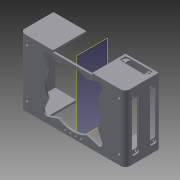
# Autodesk Inventor part: Enclosure03
Saved by Autodesk Inventor 2013 (Build 170138000, 138)
## iProperties
Created: 2014-04-13
Part Number: Enclosure03
Material: Generic
Document SubType Name: Modeling
Designer: spichelh
Density: 1 g/cm^3
Author: spichelh
Autodesk Inventor part; units mm, degrees
ref_plane "YZ Plane" through (0, 0, 0) normal (1, 0, 0) x (0, 1, 0)
ref_plane "XZ Plane" through (0, 0, 0) normal (0, 1, 0) x (-1, 0, 0)
ref_plane "XY Plane" through (0, 0, 0) normal (0, 0, 1) x (1, 0, 0)
sketch "Sketch1" plane through (0, 0, 0) normal (0, 0, 1) x (1, 0, 0)
  circle A0 centre (31.4469, 31.0185) radius 28
  line L0 (-19.3531, 19.1035) -> (82.2469, 19.1035) construction
  line L1 (8.064, 76.2535) -> (-19.3531, 76.2535) construction
  line L2 (82.2469, 76.2535) -> (53.944, 76.2535) construction
  line L3 (82.2469, 19.1035) -> (82.2469, 76.2535) construction
  line L4 (-19.3531, 76.2535) -> (-19.3531, 19.1035) construction
  circle A1 centre (5.126, 22.9135) radius 1.5 construction
  line L5 (5.509, -3.7465) -> (61.389, -3.7465) construction
  line L6 (-22.3531, -3.7465) -> (85.2469, -3.7465)
  line L7 (85.2469, -3.7465) -> (85.2469, 64.2535)
  line L8 (31.4469, -3.7465) -> (31.4469, 78.2535) construction
  circle A2 centre (31.4469, 31.0185) radius 23 projected
  line L9 (-22.3531, 64.2535) -> (-22.3531, -3.7465)
  line L10 (-22.3531, 64.2535) -> (85.2469, 64.2535)
  point P0 (0, 0)
  dimension "d42" = 0
  dimension "d44" = 3
  dimension "d47" = 57.15
  dimension "d49" = 101.6
  dimension "d50" = 3.81
  dimension "d59" = 56
  dimension "d199" = 68
  dimension "d202" = 107.6
  dimension "d374" = 3.7465
  dimension "d375" = 22.3531
  constraints: 22 end point, 2 centre point, 2 parallel, 1 concentric, 1 horizontal, 1 midpoint, 1 perpendicular, 1 point on line, 1 symmetric about line
  measures "d42" distance between parallel lines of L6 L5
  measures "d44" distance between parallel lines of L7 L3
  measures "d47" distance between parallel lines of L0 L1
  measures "d49" distance between parallel lines of L4 L3
  measures "d50" distance from line of L0 A1.centre
  measures "d59" diameter of A0
  measures "d199" distance of L9.start L6.start
  measures "d202" distance between parallel lines of L9 L7
  measures "d374" distance from line of L6 point (0, 0)
  measures "d375" distance from line of L9 point (0, 0)
extrude "Extrusion1" add sketch "Sketch1" along normal blind 2 contours A0 | L9 L10 L7 L6
sketch "Sketch4" plane through (0, 0, 2) normal (0, 0, 1) x (1, 0, 0)
  circle A0 centre (-15.5431, 55.7835) radius 1.5 projected
  circle A1 centre (-15.5431, 6.2535) radius 1.5 projected
  circle A2 centre (78.4369, 6.2535) radius 1.5 projected
  circle A3 centre (78.4369, 55.7835) radius 1.5 projected
  circle A4 centre (-15.5431, 55.7835) radius 1.4
  circle A5 centre (-15.5431, 6.2535) radius 1.4
  circle A6 centre (78.4369, 6.2535) radius 1.4
  circle A7 centre (78.4369, 55.7835) radius 1.4
  point P0 (0, 0)
  dimension "d490" = 2.8
  dimension "d491" = 2.8
  dimension "d492" = 2.8
  dimension "d493" = 2.8
  constraints: 4 centre point, 4 coincident
  measures "d490" diameter of A4
  measures "d491" diameter of A5
  measures "d492" diameter of A6
  measures "d493" diameter of A7
extrude "Extrusion3" cut sketch "Sketch4" against normal blind 10 contours A4 | A5 | A6 | A7
sketch "Sketch2" plane through (0, 0, 0) normal (0, 0, -1) x (-1, 0, 0)
  circle A0 centre (-31.4469, 31.0185) radius 23 projected
  line L0 (20.3531, 62.2535) -> (20.3531, -1.7465)
  line L1 (20.3531, -1.7465) -> (-83.2469, -1.7465)
  line L2 (-83.2469, -1.7465) -> (-83.2469, 62.2535)
  line L3 (-83.2469, 62.2535) -> (20.3531, 62.2535)
  circle A1 centre (-31.4469, 31.0185) radius 23 projected
  line L4 (22.3531, -3.7465) -> (-85.2469, -3.7465) projected
  line L5 (22.3531, 64.2535) -> (22.3531, -3.7465) projected
  line L6 (-85.2469, 64.2535) -> (22.3531, 64.2535) projected
  line L7 (-85.2469, -3.7465) -> (-85.2469, 64.2535) projected
  dimension "d454" = 2
  dimension "d455" = 2
  dimension "d456" = 2
  dimension "d457" = 2
  constraints: 8 end point
  measures "d454" distance between parallel lines of L6 L3
  measures "d455" distance between parallel lines of L5 L0
  measures "d456" distance between parallel lines of L4 L1
  measures "d457" distance between parallel lines of L7 L2
extrude "Extrusion2" add sketch "Sketch2" along normal blind 32 contours L4 L7 L6 L5
ref_plane "Work Plane1" through (0, 0, 7) normal (0, 0, -1) x (-1, 0, 0)
sketch "Sketch28" plane through (0, 0, 7) normal (0, 0, -1) x (-1, 0, 0)
  circle A0 centre (-31.4469, 31.0185) radius 28 projected
  circle A1 centre (-31.4469, 31.0185) radius 31
  point P0 (0, 0)
  dimension "d209" = 62
  constraints: 1 centre point, 1 coincident
  measures "d209" diameter of A1
extrude "Extrusion23" [suppressed]
sketch "Sketch5" plane through (-22.3531, 77.2535, 10) normal (0, 1, 0) x (-0.9933511, 0, -0.1151242)
  line L0 (0, 0) -> (128.1647, 0)
  line L1 (36.0824, 63) -> (92.0824, 63)
  line L2 (92.0824, 63) -> (92.0824, 7)
  line L3 (92.0824, 7) -> (36.0824, 7)
  line L4 (36.0824, 7) -> (36.0824, 63)
  line L5 (64.0824, 0) -> (64.0824, -31.7336) construction
  line L6 (36.0824, 63) -> (92.0824, 7) construction
  line L7 (92.0824, 63) -> (36.0824, 7) construction
  line L8 (104.9242, 0) -> (-0.6758, 0)
  line L9 (-53.8, -48) -> (-9.5691, -16.8574) construction
  point P0 (19.351, -30)
  point P1 (64.0824, 35)
  point P2 (64.0824, 35)
  dimension "d28" = 56
  dimension "d29" = 56
  dimension "d41" = 7
  constraints: 20 end point, 3 midpoint, 3 parallel, 2 point on line, 1 collinear, 1 horizontal, 1 perpendicular
  measures "d28" distance of L2.end L3.end
  measures "d29" distance of L1.end L2.end
  measures "d41" distance between parallel lines of L8 L3
extrude "Extrusion4" [suppressed]
sketch "Sketch6" plane through (-6.7798, 80.573, 3) normal (0, 1, 0) x (1, 0, 0)
  line L0 (71.5763, -7) -> (-25.8, -7) projected
  line L1 (0, 0) -> (56, 0)
  line L2 (56, 0) -> (56, -7)
  line L3 (56, -7) -> (0, -7)
  line L4 (0, -7) -> (0, 0)
  point P0 (76.8, -7)
  point P1 (-20.8, -7)
  point P2 (6.7798, 3)
  point P3 (71.5763, -8)
  point P4 (-25.8, -7)
  constraints: 8 end point, 2 parallel, 1 horizontal, 1 perpendicular, 2 other
extrude "Extrusion5" [suppressed]
sketch "Sketch7" plane through (0, 0, 2) normal (0, 0, 1) x (1, 0, 0)
  line L0 (-22.3531, -3.7465) -> (85.2469, -3.7465) projected
  line L1 (59.4469, 75.7535) -> (3.4469, 75.7535) projected
  line L2 (31.4469, -3.7465) -> (31.4469, 75.7535) construction
  line L3 (23.1969, -0.7465) -> (23.1969, -0.7465)
  line L4 (22.1969, 0.2535) -> (22.1969, 1.2535)
  line L5 (23.1969, 2.2535) -> (23.1969, 2.2535)
  line L6 (24.1969, 1.2535) -> (24.1969, 0.2535)
  arc A0 (24.1969, 1.2535) -> (23.1969, 2.2535) centre (23.1969, 1.2535) ccw
  arc A1 (23.1969, 2.2535) -> (22.1969, 1.2535) centre (23.1969, 1.2535) ccw
  arc A2 (22.1969, 0.2535) -> (23.1969, -0.7465) centre (23.1969, 0.2535) ccw
  arc A3 (23.1969, -0.7465) -> (24.1969, 0.2535) centre (23.1969, 0.2535) ccw
  line L7 (27.6969, 0.2535) -> (27.6969, 1.2535)
  line L8 (29.6969, 1.2535) -> (29.6969, 0.2535)
  arc A4 (29.6969, 1.2535) -> (28.6969, 2.2535) centre (28.6969, 1.2535) ccw
  arc A5 (28.6969, 2.2535) -> (27.6969, 1.2535) centre (28.6969, 1.2535) ccw
  arc A6 (27.6969, 0.2535) -> (28.6969, -0.7465) centre (28.6969, 0.2535) ccw
  arc A7 (28.6969, -0.7465) -> (29.6969, 0.2535) centre (28.6969, 0.2535) ccw
  line L9 (33.1969, 0.2535) -> (33.1969, 1.2535)
  line L10 (35.1969, 1.2535) -> (35.1969, 0.2535)
  arc A8 (35.1969, 1.2535) -> (34.1969, 2.2535) centre (34.1969, 1.2535) ccw
  arc A9 (34.1969, 2.2535) -> (33.1969, 1.2535) centre (34.1969, 1.2535) ccw
  arc A10 (33.1969, 0.2535) -> (34.1969, -0.7465) centre (34.1969, 0.2535) ccw
  arc A11 (34.1969, -0.7465) -> (35.1969, 0.2535) centre (34.1969, 0.2535) ccw
  line L11 (38.6969, 0.2535) -> (38.6969, 1.2535)
  line L12 (40.6969, 1.2535) -> (40.6969, 0.2535)
  arc A12 (40.6969, 1.2535) -> (39.6969, 2.2535) centre (39.6969, 1.2535) ccw
  arc A13 (39.6969, 2.2535) -> (38.6969, 1.2535) centre (39.6969, 1.2535) ccw
  arc A14 (38.6969, 0.2535) -> (39.6969, -0.7465) centre (39.6969, 0.2535) ccw
  arc A15 (39.6969, -0.7465) -> (40.6969, 0.2535) centre (39.6969, 0.2535) ccw
  line L13 (29.6969, 0.7535) -> (33.1969, 0.7535) construction
  point P0 (-17.3531, -3.7465)
  point P1 (80.2469, -3.7465)
  point P2 (0, 0)
  point P3 (24.1969, -0.7465)
  point P4 (22.1969, 2.2535)
  point P5 (24.1969, 2.2535)
  point P6 (29.6969, -0.7465)
  point P7 (27.6969, 2.2535)
  point P8 (29.6969, 2.2535)
  point P9 (35.1969, -0.7465)
  point P10 (33.1969, 2.2535)
  point P11 (35.1969, 2.2535)
  point P12 (40.6969, -0.7465)
  point P13 (38.6969, 2.2535)
  point P14 (40.6969, 2.2535)
  point P15 (31.4469, 0.7535)
  dimension "d64" = 2
  dimension "d66" = 3
  dimension "d67" = 1
  dimension "d68" = 1
  dimension "d69" = 4
  dimension "d78" = 16.5
  dimension "d79" = 7.25
  dimension "d80" = 7.25
  constraints: 32 point on circle, 24 end point, 16 centre point, 16 point on line, 8 tangent, 5 midpoint, 2 equal radius, 2 parallel, 1 horizontal, 1 perpendicular
  measures "d64" distance of point (22.197, 2.253) point (24.197, 2.253)
  measures "d66" distance of point (24.197, 2.253) point (24.197, -0.747)
  measures "d67" radius of A0
  measures "d68" radius of A3
  measures "d69" distance from line of L0 A3.centre
  measures "d78" distance of A14.centre A3.centre
  measures "d79" distance from line of L6 point (31.447, 0.753)
  measures "d80" distance from line of point (31.447, 0.753) L11
extrude "Extrusion6" cut sketch "Sketch7" against normal blind 5
sketch "Sketch42" plane through (0, 0, 2) normal (0, 0, 1) x (1, 0, 0)
  circle A0 centre (31.4469, 31.0185) radius 28 projected
  arc A1 (33.1969, 0.2535) -> (35.1969, 0.2535) centre (34.1969, 0.2535) ccw projected
  line L0 (33.1969, 0.2535) -> (33.1969, 1.2535) projected
  arc A2 (35.1969, 1.2535) -> (33.1969, 1.2535) centre (34.1969, 1.2535) ccw projected
  line L1 (35.1969, 1.2535) -> (35.1969, 0.2535) projected
  arc A3 (33.1969, 0.2535) -> (35.1969, 0.2535) centre (34.1969, 0.2535) ccw projected
  circle A4 centre (31.4469, 27.6995) radius 31 projected
  line L2 (38.6969, 0.2535) -> (38.6969, 1.2535) projected
  arc A5 (40.6969, 1.2535) -> (38.6969, 1.2535) centre (39.6969, 1.2535) ccw projected
  circle A6 centre (31.4469, 27.6995) radius 31 projected
  arc A7 (24.1969, 1.2535) -> (22.1969, 1.2535) centre (23.1969, 1.2535) ccw projected
  line L3 (24.1969, 1.2535) -> (24.1969, 0.2535) projected
  circle A8 centre (31.4469, 27.6995) radius 31 projected
  arc A9 (27.6969, 0.2535) -> (29.6969, 0.2535) centre (28.6969, 0.2535) ccw projected
  line L4 (27.6969, 0.2535) -> (27.6969, 1.2535) projected
  arc A10 (29.6969, 1.2535) -> (27.6969, 1.2535) centre (28.6969, 1.2535) ccw projected
  line L5 (29.6969, 1.2535) -> (29.6969, 0.2535) projected
  arc A11 (27.6969, 0.2535) -> (29.6969, 0.2535) centre (28.6969, 0.2535) ccw projected
  circle A12 centre (31.4469, 27.6995) radius 31 projected
  point P0 (33.214, 0.0694)
  point P1 (35.1969, 0.2466)
  point P2 (38.6969, 0.8787)
  point P3 (40.6819, 1.4265)
  point P4 (22.212, 1.4265)
  point P5 (24.1969, 0.8787)
  point P6 (27.697, 0.2466)
  point P7 (29.6799, 0.0694)
  point P8 (0, 0)
  point P9 (33.2141, 0.0689)
  point P10 (35.1969, 0.2461)
  point P11 (38.6969, 0.8782)
  point P12 (40.6819, 1.426)
  point P13 (22.2119, 1.426)
  point P14 (24.1969, 0.8782)
  point P15 (27.697, 0.2461)
  point P16 (29.6798, 0.0689)
  constraints: 1 coincident, 4 other
sketch "Sketch43" plane through (0, 0, 2) normal (0, 0, 1) x (1, 0, 0)
  circle A0 centre (4.7769, 55.7835) radius 1.4
  arc A1 (5.8515, 59.1144) -> (1.5346, 54.4655) centre (4.7769, 55.7835) ccw
  circle A2 centre (31.4469, 31.0185) radius 20
  line L0 (5.8515, 59.1144) -> (16.9262, 55.5419)
  line L1 (1.5346, 54.4655) -> (5.9166, 43.6854)
  circle A3 centre (4.7769, 6.2535) radius 1.4
  circle A4 centre (58.1169, 6.2535) radius 1.4
  line L2 (58.1169, 55.7835) -> (4.7769, 6.2535) construction
  line L3 (58.1169, 6.2535) -> (4.7769, 55.7835) construction
  line L4 (31.4469, 31.0185) -> (31.4469, 40.8752) construction
  line L5 (31.4469, 31.0185) -> (19.6856, 31.0185) construction
  line L6 (57.0424, 59.1144) -> (45.9677, 55.5419)
  arc A5 (61.3593, 54.4655) -> (57.0424, 59.1144) centre (58.1169, 55.7835) ccw
  line L7 (61.3593, 54.4655) -> (56.9773, 43.6854)
  circle A6 centre (58.1169, 55.7835) radius 1.4
  arc A7 (45.9677, 55.5419) -> (16.9262, 55.5419) centre (31.4469, 31.0185) ccw
  arc A8 (5.9166, 43.6854) -> (56.9773, 43.6854) centre (31.4469, 31.0185) ccw construction
  arc A9 (45.9677, 55.5419) -> (16.9262, 55.5419) centre (31.4469, 31.0185) ccw construction
  arc A10 (1.5346, 7.5715) -> (5.8515, 2.9225) centre (4.7769, 6.2535) ccw
  line L8 (5.8515, 2.9225) -> (16.9262, 6.495)
  line L9 (1.5346, 7.5715) -> (5.9166, 18.3516)
  line L10 (61.3593, 7.5715) -> (56.9773, 18.3516)
  arc A11 (57.0424, 2.9225) -> (61.3593, 7.5715) centre (58.1169, 6.2535) ccw
  line L11 (57.0424, 2.9225) -> (45.9677, 6.495)
  arc A12 (56.9773, 18.3516) -> (56.9773, 43.6854) centre (31.4469, 31.0185) ccw
  arc A13 (5.9166, 43.6854) -> (5.9166, 18.3516) centre (31.4469, 31.0185) ccw
  arc A14 (16.9262, 6.495) -> (45.9677, 6.495) centre (31.4469, 31.0185) ccw
  circle A15 centre (31.4469, 31.0185) radius 28 projected
  line L12 (85.2469, -1.7465) -> (85.2469, 65.2535) construction
  line L13 (85.2469, 65.2535) -> (54.4469, 65.2535) construction
  line L14 (8.4469, 65.2535) -> (-22.3531, 65.2535) construction
  line L15 (-22.3531, 65.2535) -> (-22.3531, -1.7465) construction
  line L16 (-20.3531, -3.7465) -> (83.2469, -3.7465) construction
  line L17 (85.2469, 65.2535) -> (-22.0418, -2.818) construction
  line L18 (-22.3531, 65.2535) -> (84.9357, -2.818) construction
  point P0 (3.5014, 0.0834)
  point P1 (31.4469, 31.0185)
  point P2 (67.9135, 65.2535)
  point P3 (-5.0196, 65.2535)
  point P4 (-10.4012, -3.7465)
  point P5 (73.2951, -3.7465)
  dimension "d345" = 2.8
  dimension "d346" = 7
  dimension "d347" = 40
  dimension "d348" = 27.9456
  dimension "d349" = 53.34
  dimension "d350" = 49.53
  dimension "d351" = 2.8
  dimension "d352" = 2.8
  dimension "d353" = 155
  dimension "d354" = 155
  dimension "d355" = 30.9351
  dimension "d356" = 28.5
  dimension "d357" = 155
  dimension "d358" = 3.5
  dimension "d359" = 155
  dimension "d360" = 28.5
  constraints: 28 end point, 22 point on circle, 15 centre point, 10 symmetric about line, 7 coincident, 4 tangent, 2 horizontal alignment, 2 midpoint, 2 vertical alignment, 1 perpendicular, 9 other
  measures "d345" diameter of A0
  measures "d346" diameter of A1
  measures "d347" diameter of A2
  measures "d348" horizontal distance of L4.start point (3.501, 0.083)
  measures "d349" distance of A0.centre L2.start
  measures "d350" distance of point (4.777, 6.253) A0.centre
  measures "d351" diameter of A3
  measures "d352" diameter of A4
  measures "d353" angle of L3 L0
  measures "d354" angle of L3 L1
  measures "d355" vertical distance of point (3.501, 0.083) A8.centre
  measures "d356" radius of A7
  measures "d357" angle of L8 L2
  measures "d358" radius of A10
  measures "d359" angle of L2 L9
  measures "d360" radius of A12
extrude "Extrusion32" cut sketch "Sketch43" against normal blind 10 contours A0 | L0 A7 L6 A5 L7 A12 L10 A11 L11 A14 L8 A10 L9 A13 L1 A1 | A3 | A4 | A6 | A15
sketch "Sketch44" plane through (85.2469, -3.7465, 2) normal (1, 0, 0) x (0, 0, -1)
  line L0 (9, 56.4) -> (12, 56.4)
  line L1 (14, 54.4) -> (14, 13.4)
  line L2 (12, 11.4) -> (9, 11.4)
  line L3 (7, 13.4) -> (7, 54.4)
  line L4 (10.671, 0) -> (39, 0)
  arc A0 (14, 54.4) -> (12, 56.4) centre (12, 54.4) ccw
  arc A1 (9, 56.4) -> (7, 54.4) centre (9, 54.4) ccw
  arc A2 (12, 11.4) -> (14, 13.4) centre (12, 13.4) ccw
  arc A3 (7, 13.4) -> (9, 11.4) centre (9, 13.4) ccw
  line L5 (0, 0) -> (0, 68) projected
  line L6 (34, 0) -> (0, 0) projected
  line L7 (34, 68) -> (0, 68) projected
  line L8 (0, 0) -> (0, 68) projected
  line L9 (34, 0) -> (0, 0) projected
  line L10 (34, 68) -> (34, 0) projected
  point P0 (-28, 1.7465)
  point P1 (7, 56.4)
  point P2 (14, 56.4)
  point P3 (-39, 45.4825)
  point P4 (-57, 11.6532)
  point P5 (0, 15.1877)
  point P6 (0, 0)
  dimension "d310" = 45
  dimension "d312" = 7
  dimension "d313" = 11.4
  dimension "d314" = 7
  dimension "d315" = 2
  dimension "d483" = 11.6
  constraints: 10 end point, 8 point on circle, 8 tangent, 5 point on line, 4 centre point, 3 equal radius, 2 parallel, 1 collinear, 1 horizontal, 1 perpendicular, 4 other
  measures "d310" distance between parallel lines of L0 L2
  measures "d312" distance of point (7, 56.4) point (14, 56.4)
  measures "d313" distance between parallel lines of L4 L2
  measures "d314" distance of the line from the sketch origin of L3
  measures "d315" radius of A0
  measures "d483" distance between parallel lines of L7 L0
extrude "Extrusion33" cut sketch "Sketch44" against normal blind 50 contours L0 A0 L1 A2 L2 A3 L3 A1
sketch "Sketch45" plane through (85.2469, -3.7465, 2) normal (1, 0, 0) x (0, 0, -1)
  arc A0 (9, 56.4) -> (7, 54.4) centre (9, 54.4) ccw
  line L0 (9, 56.4) -> (12, 56.4)
  arc A1 (14, 54.4) -> (12, 56.4) centre (12, 54.4) ccw
  line L1 (14, 54.4) -> (14, 13.4)
  arc A2 (12, 11.4) -> (14, 13.4) centre (12, 13.4) ccw
  line L2 (12, 11.4) -> (9, 11.4)
  arc A3 (7, 13.4) -> (9, 11.4) centre (9, 13.4) ccw
  line L3 (7, 13.4) -> (7, 54.4)
  line L4 (9, 60.4) -> (12, 60.4)
  line L5 (14, 58.4) -> (14, 9.4)
  line L6 (12, 7.4) -> (9, 7.4)
  line L7 (7, 9.4) -> (7, 58.4)
  arc A4 (14, 58.4) -> (12, 60.4) centre (12, 58.4) ccw
  arc A5 (9, 60.4) -> (7, 58.4) centre (9, 58.4) ccw
  arc A6 (12, 7.4) -> (14, 9.4) centre (12, 9.4) ccw
  arc A7 (7, 9.4) -> (9, 7.4) centre (9, 9.4) ccw
  arc A8 (9, 56.4) -> (7, 54.4) centre (9, 54.4) ccw projected
  line L8 (9, 56.4) -> (12, 56.4) projected
  line L9 (12, 11.4) -> (9, 11.4) projected
  arc A9 (7, 13.4) -> (9, 11.4) centre (9, 13.4) ccw projected
  line L10 (7, 13.4) -> (7, 54.4) projected
  arc A10 (14, 54.4) -> (12, 56.4) centre (12, 54.4) ccw projected
  line L11 (14, 54.4) -> (14, 13.4) projected
  arc A11 (12, 11.4) -> (14, 13.4) centre (12, 13.4) ccw projected
  point P0 (-28, 1.7465)
  point P1 (-29.2165, 54.9882)
  point P2 (-29.1727, 10.0075)
  dimension "d485" = 2
  dimension "d487" = 2
  dimension "d330" = 0
  dimension "d331" = 4
  dimension "d332" = 4
  dimension "d333" = 0
  dimension "d334" = 2
  dimension "d484" = 2
  dimension "d486" = 2
  dimension "d488" = 2
  constraints: 16 end point, 12 point on circle, 8 tangent, 6 centre point, 4 coincident, 4 collinear, 3 equal radius, 2 parallel, 1 horizontal, 1 perpendicular, 8 other
  measures "d330" distance between parallel lines of L5 L1
  measures "d331" distance between parallel lines of L4 L0
  measures "d332" distance between parallel lines of L2 L6
  measures "d333" distance between parallel lines of L3 L7
  measures "d334" radius of A4
  measures "d484" radius of A2
  measures "d486" radius of A6
  measures "d488" radius of A1
extrude "Extrusion34" cut sketch "Sketch45" against normal blind 1.5 contours A0 L7 A5 L4 A4 L5 A1 L0 | A3 L2 A2 L5 A6 L6 A7 L7
sketch "Sketch46" plane through (85.2469, -3.7465, 2) normal (1, 0, 0) x (0, 0, -1)
  line L0 (12, 56.4) -> (9, 56.4)
  line L1 (-25, 13.4) -> (-25, 54.4)
  arc A0 (9, 60.4) -> (7, 58.4) centre (9, 58.4) ccw
  line L2 (14, 58.4) -> (14, 9.4)
  circle A1 centre (9, 58.4) radius 1
  line L3 (9, 58.4) -> (7.5858, 59.8142) construction
  line L4 (10.5, 56.4) -> (10.5, 46.2799) construction
  circle A2 centre (12, 58.4) radius 1
  line L5 (-25, 33.9) -> (-40, 33.9) construction
  circle A3 centre (9, 9.4) radius 1
  circle A4 centre (12, 9.4) radius 1
  line L6 (12, 56.4) -> (9, 56.4) projected
  arc A5 (9, 60.4) -> (7, 58.4) centre (9, 58.4) ccw projected
  arc A6 (12, 7.4) -> (14, 9.4) centre (12, 9.4) ccw projected
  point P0 (2, 3.7465)
  point P1 (-29.1529, 58.9941)
  dimension "d337" = 2
  dimension "d340" = 0
  constraints: 12 end point, 4 centre point, 3 symmetric about line, 2 coincident, 2 midpoint, 1 collinear, 1 parallel, 1 perpendicular, 1 point on line, 8 other
  measures "d337" diameter of A1
  measures "d340" distance of L3.start A1.centre
extrude "Extrusion35" cut sketch "Sketch46" against normal blind 2 contours A1 | A4
fillet "Fillet12" radius 0.2 9 edges at (59.1683, 49.0754, 2) (59.9469, 31.0185, 2) (59.1683, 12.9615, 2) (31.4469, 2.5185, 2) (51.505, 4.7088, 2) (11.3888, 4.7088, 2) (3.7256, 12.9615, 2) (2.9469, 31.0185, 2) (3.7256, 49.0754, 2)
fillet "Fillet13" radius 0.2 14 edges at (85.2469, 4.2393, -11.4142) (85.2469, 3.6535, -8.5) (85.2469, 4.2393, -5.5858) (85.2469, 30.1535, -5) (85.2469, 56.0677, -5.5858) (85.2469, 56.6535, -8.5) (85.2469, 56.0677, -11.4142) (85.2469, 30.1535, -12) (83.7469, 52.0677, -11.4142) (83.7469, 52.6535, -8.5) (83.7469, 52.0677, -5.5858) (83.7469, 8.2393, -5.5858) (83.7469, 7.6535, -8.5) (83.7469, 8.2393, -11.4142)
sketch "Sketch50" plane through (85.2469, -3.7465, 2) normal (1, 0, 0) x (0, 0, -1)
  line L0 (0, 68) -> (-34.1358, 68)
  line L1 (0, 8) -> (0, 57)
  line L2 (27.2, 56.3) -> (30.2, 56.3)
  line L3 (32.2, 54.3) -> (32.2, 13.3)
  line L4 (30.2, 11.3) -> (27.2, 11.3)
  line L5 (25.2, 13.3) -> (25.2, 54.3)
  arc A0 (32.2, 54.3) -> (30.2, 56.3) centre (30.2, 54.3) ccw
  arc A1 (27.2, 56.3) -> (25.2, 54.3) centre (27.2, 54.3) ccw
  arc A2 (30.2, 11.3) -> (32.2, 13.3) centre (30.2, 13.3) ccw
  arc A3 (25.2, 13.3) -> (27.2, 11.3) centre (27.2, 13.3) ccw
  line L6 (34, 68) -> (0, 68) projected
  line L7 (0, 0) -> (0, 68) projected
  line L8 (34, 68) -> (34, 0) projected
  point P0 (0, 68)
  point P1 (-34.1358, 68)
  point P2 (-28, 1.7465)
  point P3 (25.2, 56.3)
  point P4 (32.2, 56.3)
  point P5 (-28.0348, 67)
  point P6 (-34, 67)
  dimension "d400" = 45
  dimension "d401" = 7
  dimension "d402" = 2
  dimension "d404" = 11.7
  dimension "d478" = 1.8
  constraints: 10 end point, 8 point on circle, 8 tangent, 4 centre point, 4 point on line, 3 equal radius, 2 horizontal, 2 parallel, 1 collinear, 1 perpendicular, 3 other
  measures "d400" distance between parallel lines of L2 L4
  measures "d401" distance of point (25.2, 56.3) point (32.2, 56.3)
  measures "d402" radius of A0
  measures "d478" distance between parallel lines of L3 L8
extrude "Extrusion39" cut sketch "Sketch50" against normal blind 5
sketch "Sketch51" plane through (85.2469, -3.7465, 2) normal (1, 0, 0) x (0, 0, -1)
  arc A0 (32.2, 54.3) -> (30.2, 56.3) centre (30.2, 54.3) ccw
  line L0 (32.2, 54.3) -> (32.2, 13.3)
  arc A1 (30.2, 11.3) -> (32.2, 13.3) centre (30.2, 13.3) ccw
  line L1 (30.2, 11.3) -> (27.2, 11.3)
  arc A2 (25.2, 13.3) -> (27.2, 11.3) centre (27.2, 13.3) ccw
  line L2 (25.2, 13.3) -> (25.2, 54.3)
  arc A3 (27.2, 56.3) -> (25.2, 54.3) centre (27.2, 54.3) ccw
  line L3 (27.2, 56.3) -> (30.2, 56.3)
  line L4 (27.2, 60.3) -> (30.2, 60.3)
  line L5 (32.2, 58.3) -> (32.2, 9.3)
  line L6 (30.2, 7.3) -> (27.2, 7.3)
  line L7 (25.2, 9.3) -> (25.2, 58.3)
  arc A4 (32.2, 58.3) -> (30.2, 60.3) centre (30.2, 58.3) ccw
  arc A5 (27.2, 60.3) -> (25.2, 58.3) centre (27.2, 58.3) ccw
  arc A6 (30.2, 7.3) -> (32.2, 9.3) centre (30.2, 9.3) ccw
  arc A7 (25.2, 9.3) -> (27.2, 7.3) centre (27.2, 9.3) ccw
  arc A8 (32.2, 54.3) -> (30.2, 56.3) centre (30.2, 54.3) ccw projected
  line L8 (30.2, 11.3) -> (27.2, 11.3) projected
  arc A9 (25.2, 13.3) -> (27.2, 11.3) centre (27.2, 13.3) ccw projected
  line L9 (25.2, 13.3) -> (25.2, 54.3) projected
  arc A10 (27.2, 56.3) -> (25.2, 54.3) centre (27.2, 54.3) ccw projected
  line L10 (27.2, 56.3) -> (30.2, 56.3) projected
  line L11 (32.2, 54.3) -> (32.2, 13.3) projected
  arc A11 (30.2, 11.3) -> (32.2, 13.3) centre (30.2, 13.3) ccw projected
  point P0 (-28, 1.7465)
  point P1 (0, 53.833)
  point P2 (0, 9.167)
  dimension "d480" = 2
  dimension "d482" = 2
  dimension "d411" = 2
  dimension "d412" = 4
  dimension "d413" = 4
  dimension "d415" = 0
  dimension "d479" = 2
  dimension "d481" = 2
  constraints: 16 end point, 12 point on circle, 8 tangent, 6 centre point, 5 collinear, 4 coincident, 3 equal radius, 2 parallel, 1 horizontal, 1 perpendicular, 1 vertical, 8 other
  measures "d411" radius of A4
  measures "d412" distance between parallel lines of L6 L1
  measures "d413" distance between parallel lines of L4 L3
  measures "d415" distance between parallel lines of L2 L7
  measures "d479" radius of A3
  measures "d481" radius of A2
extrude "Extrusion40" cut sketch "Sketch51" against normal blind 1.5 contours A0 L3 A3 L7 A5 L4 A4 L5 | L5 A6 L6 A7 L7 A2 L1 A1
fillet "Fillet16" radius 0.2 14 edges at (85.2469, 4.1393, -29.6142) (85.2469, 3.5535, -26.7) (85.2469, 4.1393, -23.7858) (85.2469, 30.0535, -23.2) (85.2469, 55.9677, -23.7858) (85.2469, 56.5535, -26.7) (85.2469, 55.9677, -29.6142) (85.2469, 30.0535, -30.2) (83.7469, 52.5535, -26.7) (83.7469, 51.9677, -23.7858) (83.7469, 8.1393, -23.7858) (83.7469, 7.5535, -26.7) (83.7469, 8.1393, -29.6142) (83.7469, 51.9677, -29.6142)
sketch "Sketch52" plane through (83.7469, -3.7465, 2) normal (1, 0, 0) x (0, 0, -1)
  arc A0 (30.2, 7.3) -> (32.2, 9.3) centre (30.2, 9.3) ccw projected
  arc A1 (27.2, 60.3) -> (25.2, 58.3) centre (27.2, 58.3) ccw projected
  circle A2 centre (27.2, 58.3) radius 1
  circle A3 centre (30.2, 9.3) radius 1
  point P0 (2, 3.7465)
  dimension "d419" = 2
  dimension "d420" = 2
  constraints: 2 centre point, 2 coincident
  measures "d419" diameter of A2
  measures "d420" diameter of A3
extrude "Extrusion41" cut sketch "Sketch52" against normal blind 2
sketch "Sketch53" plane through (-22.3531, 64.2535, 2) normal (0, 1, 0) x (1, 0, 0)
  line L0 (82.1, 32.2) -> (98.1, 32.2)
  line L1 (100.1, 30.2) -> (100.1, 27.2)
  line L2 (98.1, 25.2) -> (82.1, 25.2)
  line L3 (80.1, 27.2) -> (80.1, 30.2)
  arc A0 (82.1, 32.2) -> (80.1, 30.2) centre (82.1, 30.2) ccw
  arc A1 (80.1, 27.2) -> (82.1, 25.2) centre (82.1, 27.2) ccw
  arc A2 (98.1, 25.2) -> (100.1, 27.2) centre (98.1, 27.2) ccw
  arc A3 (100.1, 30.2) -> (98.1, 32.2) centre (98.1, 30.2) ccw
  line L4 (107.6, 34) -> (107.6, 0) projected
  line L5 (0, 34) -> (107.6, 34) projected
  point P0 (-54.4469, -28)
  point P1 (30.8, -28.0348)
  point P2 (30.8, -34)
  dimension "d423" = 7
  dimension "d425" = 2
  dimension "d426" = 20
  dimension "d460" = 7.5
  dimension "d467" = 1.8
  constraints: 8 end point, 8 point on circle, 8 tangent, 4 centre point, 3 equal radius, 2 parallel, 1 horizontal, 1 perpendicular
  measures "d423" distance between parallel lines of L2 L0
  measures "d425" radius of A0
  measures "d426" distance between parallel lines of L3 L1
  measures "d460" distance between parallel lines of L1 L4
  measures "d467" distance between parallel lines of L5 L0
extrude "Extrusion42" cut sketch "Sketch53" against normal blind 10
sketch "Sketch54" plane through (-22.3531, 64.2535, 2) normal (0, 1, 0) x (1, 0, 0)
  arc A0 (82.1, 32.2) -> (80.1, 30.2) centre (82.1, 30.2) ccw
  line L0 (82.1, 32.2) -> (98.1, 32.2)
  arc A1 (100.1, 30.2) -> (98.1, 32.2) centre (98.1, 30.2) ccw
  line L1 (100.1, 30.2) -> (100.1, 27.2)
  arc A2 (98.1, 25.2) -> (100.1, 27.2) centre (98.1, 27.2) ccw
  line L2 (98.1, 25.2) -> (82.1, 25.2)
  arc A3 (80.1, 27.2) -> (82.1, 25.2) centre (82.1, 27.2) ccw
  line L3 (80.1, 27.2) -> (80.1, 30.2)
  line L4 (78.1, 32.2) -> (102.1, 32.2)
  line L5 (104.1, 30.2) -> (104.1, 27.2)
  line L6 (102.1, 25.2) -> (78.1, 25.2)
  line L7 (76.1, 27.2) -> (76.1, 30.2)
  arc A4 (104.1, 30.2) -> (102.1, 32.2) centre (102.1, 30.2) ccw
  arc A5 (102.1, 25.2) -> (104.1, 27.2) centre (102.1, 27.2) ccw
  arc A6 (76.1, 27.2) -> (78.1, 25.2) centre (78.1, 27.2) ccw
  arc A7 (78.1, 32.2) -> (76.1, 30.2) centre (78.1, 30.2) ccw
  arc A8 (82.1, 32.2) -> (80.1, 30.2) centre (82.1, 30.2) ccw projected
  line L8 (82.1, 32.2) -> (98.1, 32.2) projected
  arc A9 (100.1, 30.2) -> (98.1, 32.2) centre (98.1, 30.2) ccw projected
  line L9 (100.1, 30.2) -> (100.1, 27.2) projected
  arc A10 (98.1, 25.2) -> (100.1, 27.2) centre (98.1, 27.2) ccw projected
  line L10 (98.1, 25.2) -> (82.1, 25.2) projected
  arc A11 (80.1, 27.2) -> (82.1, 25.2) centre (82.1, 27.2) ccw projected
  line L11 (80.1, 27.2) -> (80.1, 30.2) projected
  point P0 (-54.4469, -28)
  dimension "d431" = 2
  dimension "d432" = 4
  dimension "d433" = 4
  dimension "d462" = 2
  dimension "d463" = 2
  dimension "d464" = 2
  dimension "d465" = 2
  constraints: 16 end point, 16 point on circle, 8 centre point, 8 tangent, 6 collinear, 4 coincident, 3 equal radius, 2 horizontal, 2 parallel, 1 perpendicular
  measures "d431" radius of A4
  measures "d432" distance between parallel lines of L1 L5
  measures "d433" distance between parallel lines of L3 L7
  measures "d462" radius of A1
  measures "d463" radius of A3
  measures "d464" radius of A0
  measures "d465" radius of A2
extrude "Extrusion43" cut sketch "Sketch54" against normal blind 1.5 contours A0 L3 A3 L6 A6 L7 A7 L4 | L4 A4 L5 A5 L6 A2 L1 A1
sketch "Sketch55" plane through (-22.3531, 62.7535, 2) normal (0, 1, 0) x (1, 0, 0)
  arc A0 (104.1, 30.2) -> (102.1, 32.2) centre (102.1, 30.2) ccw projected
  circle A1 centre (102.1, 30.2) radius 1
  arc A2 (80.1, 27.2) -> (82.1, 25.2) centre (82.1, 27.2) ccw projected
  line L0 (80.1, 30.2) -> (80.1, 27.2) projected
  arc A3 (82.1, 32.2) -> (80.1, 30.2) centre (82.1, 30.2) ccw projected
  line L1 (78.1, 32.2) -> (82.1, 32.2) projected
  arc A4 (78.1, 32.2) -> (76.1, 30.2) centre (78.1, 30.2) ccw projected
  line L2 (76.1, 27.2) -> (76.1, 30.2) projected
  arc A5 (76.1, 27.2) -> (78.1, 25.2) centre (78.1, 27.2) ccw projected
  line L3 (82.1, 25.2) -> (78.1, 25.2) projected
  circle A6 centre (78.1, 27.2) radius 1
  point P0 (22.3531, 2)
  dimension "d78" = 16.5
  dimension "d79" = 7.25
  dimension "d80" = 7.25
  dimension "d436" = 2
  dimension "d437" = 2
  constraints: 2 centre point, 2 coincident
  measures "d436" diameter of A1
  measures "d437" diameter of A6
extrude "Extrusion44" cut sketch "Sketch55" against normal blind 2 contours A1 | A6
fillet "Fillet19" radius 0.2 16 edges at (24.1969, 0.7535, 2) (23.1969, -0.7465, 2) (22.1969, 0.7535, 2) (23.1969, 2.2535, 2) (29.6969, 0.7535, 2) (28.6969, -0.7465, 2) (27.6969, 0.7535, 2) (28.6969, 2.2535, 2) (35.1969, 0.7535, 2) (34.1969, -0.7465, 2) (33.1969, 0.7535, 2) (34.1969, 2.2535, 2) (40.6969, 0.7535, 2) (39.6969, -0.7465, 2) (38.6969, 0.7535, 2) (39.6969, 2.2535, 2)
fillet "Fillet22" [suppressed]
fillet "Fillet23" radius 0.3 6 edges at (85.2469, 64.2535, -15) (31.4469, 64.2535, 2) (-22.3531, 64.2535, -15) (85.2469, -3.7465, -15) (31.4469, -3.7465, 2) (-22.3531, -3.7465, -15)
fillet "Fillet24" radius 5 8 edges at (-22.2652, -3.6587, 1.9121) (-22.2652, 64.1656, 1.9121) (-22.3531, 30.2535, 2) (85.1591, 64.1656, 1.9121) (85.1591, -3.6587, 1.9121) (85.2469, 30.2535, 2) (83.2469, 30.2535, 0) (-20.3531, 30.2535, 0)
sketch "Sketch56" plane through (-20.3531, -1.7465, -32) normal (0, 1, 0) x (1, 0, 0)
  line L0 (0, 0) -> (103.6, 0) projected
  line L1 (21.63, 0) -> (81.97, 0)
  line L2 (81.97, 0) -> (81.97, -32)
  line L3 (81.97, -32) -> (21.63, -32)
  line L4 (21.63, -32) -> (21.63, 0)
  line L5 (51.8, 0) -> (51.8, -10.864) construction
  line L6 (51.8, 0) -> (51.8, -9.2141) construction
  point P0 (20.3531, -32)
  dimension "d468" = 60.34
  dimension "d470" = 32
  constraints: 12 end point, 3 parallel, 2 collinear, 2 midpoint, 1 horizontal, 1 perpendicular, 1 point on line
  measures "d468" distance between parallel lines of L2 L4
  measures "d470" distance between parallel lines of L0 L3
extrude "Extrusion45" cut sketch "Sketch56" against normal blind 10
sketch "Sketch57" plane through (-22.0531, 64.2535, -32) normal (0, 1, 0) x (1, 0, 0)
  line L0 (0, 0) -> (107, 0) projected
  line L1 (33.5, 0) -> (73.5, 0)
  line L2 (73.5, 0) -> (73.5, -40)
  line L3 (73.5, -40) -> (33.5, -40)
  line L4 (33.5, -40) -> (33.5, 0)
  line L5 (53.5, 0) -> (53.5, -7.5) construction
  line L6 (53.5, 0) -> (53.5, -19.004) construction
  point P0 (22.0531, -32)
  dimension "d473" = 40
  dimension "d475" = 40
  constraints: 12 end point, 3 parallel, 2 collinear, 2 midpoint, 1 horizontal, 1 perpendicular, 1 point on line
  measures "d473" distance between parallel lines of L2 L4
  measures "d475" distance between parallel lines of L1 L3
extrude "Extrusion46" cut sketch "Sketch57" against normal blind 2
ref_plane "Work Plane5" through (31.4469, -3.4465, -32) normal (-1, 0, 0) x (0, 0, 1)
mirror "Mirror2" about plane through (31.4469, -3.4465, -32) normal (-1, 0, 0) of "Extrusion33", "Extrusion34", "Extrusion35"
body "Solid1"
